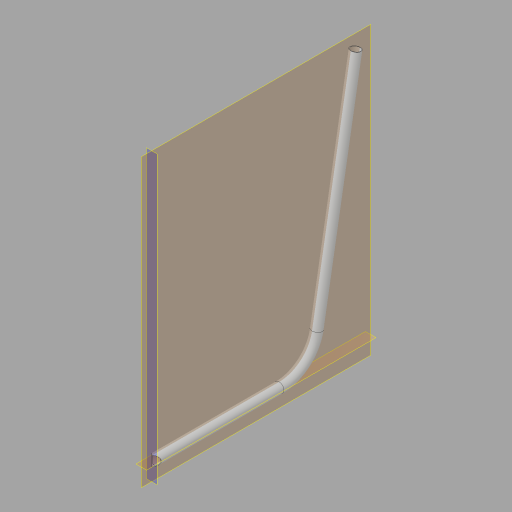
# Autodesk Inventor part: Hebel
Saved by Autodesk Inventor 2023.2 (Build 272271000, 271)
## iProperties
Created: 2023-02-02
Part Number: Hebel
Material: Generisch
Document SubType Name: Modeling
Designer: Raoul Messerli
Density: 1 g/cm^3
Appearance: Vorgabe
Author: Raoul Messerli
Autodesk Inventor part; units mm, degrees
sketch "Skizze2" plane through (0, 0, 0) normal (1, 0, 0) x (0, 1, 0)
  line L0 (0, 0) -> (1000, 0)
  arc A0 (1000, 0) -> (1295.5679, 248.6231) centre (1000, 300) ccw
  line L1 (1295.5679, 248.6231) -> (1600, 2000)
  dimension "d5" = 1000
  dimension "d6" = 300
  dimension "d7" = 1600
  dimension "d8" = 2000
  constraints: 4 end point, 2 point on circle, 2 tangent, 1 centre point, 1 coincident, 1 horizontal
  measures "d5" distance of L0.end L0.start
  measures "d6" radius of A0
  measures "d7" horizontal distance of L0.start L1.end
  measures "d8" distance from line of L1.end L0
sketch "Skizze3" plane through (0, 0, 0) normal (0, 1, 0) x (-1, 0, 0)
  circle A0 centre (0, 0) radius 38.05
  circle A1 centre (0, 0) radius 34.45
  dimension "d12" = 76.1
  dimension "d13" = 3.6
  constraints: 2 centre point, 2 coincident
  measures "d12" diameter of A0
  measures "d13" radial gap between concentric circles of A1 A0
sweep "Sweeping1" add profiles "Skizze3" path "Skizze2"
sketch "Skizze5" plane through (0, 0, 0) normal (1, 0, 0) x (0, 1, 0)
  line L0 (0, -38.05) -> (0, 38.05) projected
  circle A0 centre (0, 0) radius 38.05
  constraints: 1 coincident, 1 vertical alignment, 2 other
extrude "Extrusion3" cut sketch "Skizze5" along normal mid plane 76.1
